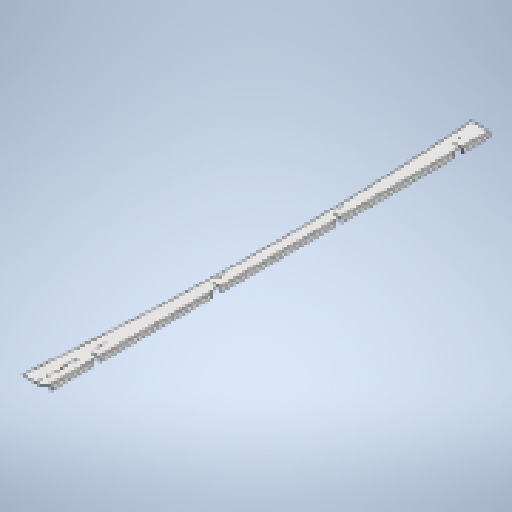
# Autodesk Inventor part: MSC 052 rib board_CPY
Saved by Autodesk Inventor 2025 (Build 290162010, 162A)
## iProperties
Created: 2024-04-28
Part Number: MSC 052 rib board_CPY
Material: Stainless Steel
Document SubType Name: Sheet Metal
Designer: admin
Stock Number: МОО 052 шпангоут борт
Density: 8 g/cm^3
Flat Pattern Width: 111.5 cm
Flat Pattern Length: 9.15826 cm
Flat Pattern Area: 1021.15 cm^2
Sheet Metal Rule: AISI304 2mm Die16
Sheet Metal Width: 1115,000 mm
Sheet Metal Length: 91,583 mm
Sheet Metal Area: 102114,551 mm^2
Appearance: Default
Author: admin
Стрингер_3: 67,524 mm
Стрингер_4: 48,201 mm
Стрингер_5: 51,522 mm
Стрингер_6: 77,509 mm
Autodesk Inventor part; units mm, degrees
note: some values were not read from the file. Chosen so that the rebuilt part matches the saved one: relief shape of "Plate4".
ref_plane "YZ Plane" through (0, 0, 0) normal (1, 0, 0) x (0, 1, 0)
ref_plane "XZ Plane" through (0, 0, 0) normal (0, 1, 0) x (-1, 0, 0)
ref_plane "XY Plane" through (0, 0, 0) normal (0, 0, 1) x (1, 0, 0)
sketch "Sketch1" plane through (0, 0, 0) normal (0, 0, 1) x (1, 0, 0)
  arc A0 (750, -2100) -> (770.156, -238.4205) centre (-10250, -1050) ccw construction
  arc A1 (752.9864, -2100.2851) -> (771.2831, -213.263) centre (-10246.9891, -1050.0292) ccw
  line L0 (-750, -2700) -> (-750, 0) construction
  line L1 (-800, 50) -> (-800, -2750) construction
  line L2 (-850, -2800) -> (-850, 100) construction
  line L3 (850, 100) -> (850, -2800)
  line L4 (800, -2750) -> (800, 50) construction
  line L5 (750, 0) -> (750, -2700) construction
  line L6 (770.156, -238.4205) -> (767.1641, -238.6409) construction
  line L7 (768.2917, -213.4901) -> (771.2831, -213.263) construction
  arc A2 (747.4657, -5.0326) -> (744.8748, -2.3426) centre (744.4792, -5.3164) ccw construction
  arc A3 (747.4657, -5.0326) -> (747.0136, -0.2851) centre (-10252.9895, -1050.2527) ccw construction
  arc A4 (767.1641, -238.6409) -> (747.4657, -5.0326) centre (-10252.9895, -1050.2527) ccw construction
  line L8 (750, 0) -> (747.0136, -0.2851) construction
  arc A5 (750.4522, -4.7486) -> (750, 0) centre (-10250, -1050) ccw construction
  arc A6 (750.4522, -4.7486) -> (745.2706, 0.6314) centre (744.4791, -5.3162) ccw
  line L9 (-750, 0) -> (750, 0) construction
  line L10 (-850, 100) -> (850, 100) construction
  line L11 (800, 50) -> (-800, 50) construction
  arc A7 (770.156, -238.4205) -> (750.4522, -4.7486) centre (-10250, -1050) ccw
  line L12 (750, -2700) -> (-750, -2700) construction
  line L13 (750, -2100) -> (752.9864, -2100.2851) construction
  line L14 (-800, -2750) -> (800, -2750)
  line L15 (850, -2800) -> (-850, -2800) construction
  arc A8 (110, -2700) -> (114.1118, -2698.3696) centre (110, -2694) ccw construction
  line L16 (0, -2697) -> (110, -2697) construction
  line L17 (0, -2700) -> (0, -2697) construction
  arc A9 (750, 0) -> (745.2706, 0.6314) centre (0, -5600) ccw construction
  line L18 (750, 0) -> (749.6018, -2.9735) construction
  arc A10 (750, -3.0268) -> (0, 47) centre (-0.2, -5603) ccw construction
  line L19 (0, 47) -> (0, 0) construction
  line L20 (0, 50) -> (0, 47) construction
  line L21 (0, 100) -> (0, 50)
  arc A11 (745.2706, 0.6314) -> (0, 50) centre (0, -5600) ccw construction
  line L22 (-750, -2100) -> (750, -2100) construction
  arc A12 (110, -2697) -> (112.0559, -2696.1848) centre (110, -2694) ccw construction
  line L23 (676.3163, -2173.4556) -> (674.2605, -2171.2708) construction
  line L24 (690.4112, -2151.9536) -> (692.4671, -2154.1384) construction
  line L25 (752.0559, -2102.1848) -> (676.3163, -2173.4556) construction
  line L26 (114.1118, -2698.3696) -> (750, -2100) construction
  arc A13 (752.0559, -2102.1848) -> (752.9864, -2100.2851) centre (749.9998, -2099.9999) ccw construction
  line L27 (750, -2100) -> (752.0559, -2102.1848) construction
  arc A14 (749.1768, -2100.7746) -> (750.1074, -2098.8746) centre (747.1209, -2098.5898) ccw construction
  line L28 (112.0559, -2696.1848) -> (690.4112, -2151.9536) construction
  line L29 (850, -258.4205) -> (774.6194, -258.4205)
  arc A15 (800, 50) -> (0, 100) centre (0, -6325) ccw construction
  arc A16 (824.6194, -258.4205) -> (800, 50) centre (-10711.2413, -1024.069) ccw construction
  line L30 (824.6194, -258.4205) -> (824.6194, 100) construction
  arc A17 (789.8132, -2131.1922) -> (824.6194, -258.4205) centre (-10201.1223, -990.2118) ccw construction
  line L31 (0, -2700) -> (0, -2750) construction
  line L32 (112.3791, -2700) -> (132.2053, -2750) construction
  line L33 (132.2053, -2750) -> (850, -2074.5565)
  arc A18 (770.0996, -238.4247) -> (766.3709, -188.564) centre (768.2917, -213.4901) ccw construction
  line L34 (850, -400) -> (783.8749, -400) construction
  line L35 (850, -900) -> (801.9923, -900) construction
  line L36 (850, -1400) -> (797.4674, -1400) construction
  line L37 (850, -1900) -> (770.2723, -1900) construction
  line L38 (350, 100) -> (350, 39.1489)
  line L39 (-1472.612, -150) -> (-973.4947, -150)
  line L40 (-1472.612, -700) -> (-973.4947, -700)
  line L41 (-1472.612, -1250) -> (-973.4947, -1250)
  line L42 (-1472.612, -1800) -> (-973.4947, -1800)
  line L43 (800, -2750) -> (850, -2750) construction
  line L44 (753.1643, -2098.4205) -> (850, -2098.4205)
  point P0 (824.6397, -2098.4205)
  dimension "d16" = 1500
  dimension "d17" = 2700
  dimension "d18" = 2100
  dimension "d19" = 6
  dimension "d20" = 3
  dimension "d21" = 3
  dimension "d22" = 6
  dimension "d23" = 3
  dimension "d24" = 239.271
  dimension "d25" = 50
  dimension "d26" = 50
  dimension "d27" = 3
  dimension "d28" = 110
  dimension "d29" = 25
  dimension "d30" = 104
  dimension "d31" = 25
  dimension "d32" = 20
  dimension "d33" = 50
  dimension "d57" = 500
  dimension "d58" = 500
  dimension "d59" = 500
  dimension "d60" = 500
  dimension "d61" = 500
  dimension "d83" = 250
  dimension "d86" = 550
  dimension "d91" = 274.5565
  dimension "d103" = 1.873
  dimension "d116" = 1840
  measures "d16" distance of L0.end L5.start
  measures "d17" distance of L5.start L5.end
  measures "d18" distance between parallel lines of L22 L9
  measures "d19" radius of A6
  measures "d20" radius of A2
  measures "d21" radius of A14
  measures "d22" radius of A8
  measures "d23" radius of A12
  measures "d24" distance of L6.start L5.start
  measures "d25" distance between parallel lines of L11 L10
  measures "d26" distance between parallel lines of L9 L11
  measures "d27" distance of L21.end L19.start
  measures "d28" distance from line of L17 A8.centre
  measures "d29" distance of L23.end L24.end
  measures "d30" distance of L27.start L23.end
  measures "d31" distance of L6.start L7.start
  measures "d32" vertical distance of L6.start L29.end
  measures "d33" distance of L30.start L29.end
  measures "d57" distance between parallel lines of L34 L10
  measures "d58" distance between parallel lines of L35 L34
  measures "d59" distance between parallel lines of L35 L36
  measures "d60" distance between parallel lines of L36 L37
  measures "d83" distance between parallel lines of L39 L10
  measures "d86" distance of L39.start L40.start
  measures "d91" distance from line of L33.end L42
  measures "d103" distance of L44.start L13.end
  measures "d116" distance between parallel lines of L44 L29
extrude "Plate3" add sketch "Sketch1" along normal blind 2 contours A1 L29 L3 L33 L44
sketch "Sketch3" plane through (848, -258.4205, 2) normal (1, 0, 0) x (0, 1, 0)
  line L0 (-1816.136, 0) -> (0, 0)
  line L1 (0, 0) -> (0, 20)
  line L2 (0, 20) -> (-1816.136, 20)
  line L3 (-1816.136, 20) -> (-1816.136, 0)
  constraints: 6 end point, 1 horizontal, 1 perpendicular, 1 vertical
edge flange "Flange2" height 20 angle 90 thickness 2 bend radius 2.75 thickness toward (1, 0, 0) relief tear relief width 2 relief depth 1 edges at (850, -1166.4885, 2) wall of the first edge with corners at (848, -2074.5565, 2) (848, -258.4205, 2) (848, -258.4205, -18) (848, -2074.5565, -18)
bend "Bend2"
corner "Corner2"
sketch "Sketch5" plane through (0, 0, 0) normal (0, 0, 1) x (1, 0, 0)
  line L0 (845.25, -2079.0263) -> (845.25, -258.4205) projected
  line L1 (774.6194, -258.4205) -> (845.25, -258.4205) projected
  arc A0 (753.1643, -2098.4205) -> (774.6194, -258.4205) centre (-10246.9891, -1050.0292) ccw projected
  line L2 (850, -258.4205) -> (850, -2074.5565) projected
  line L3 (850, -373.4205) -> (818, -373.4205)
  line L4 (850, -375.4205) -> (848, -375.4205) construction
  line L5 (848, -2074.5565) -> (848, -258.4205) projected
  line L6 (818, -373.4205) -> (818, -375.4205)
  line L7 (850, -873.4195) -> (801.5994, -873.4195) construction
  line L8 (850, -875.4195) -> (801.6312, -875.4195) construction
  line L9 (819, -873.4195) -> (819, -875.4195) construction
  line L10 (850, -1373.4195) -> (798.2777, -1373.4195) construction
  line L11 (850, -1375.4195) -> (798.2189, -1375.4195) construction
  line L12 (819, -1373.4195) -> (819, -1375.4195) construction
  line L13 (850, -1873.4195) -> (772.2907, -1873.4195) construction
  line L14 (850, -1875.4195) -> (772.1411, -1875.4195) construction
  line L15 (819, -1873.4195) -> (819, -1875.4195) construction
  line L16 (850, -904.4195) -> (845.25, -904.4195) construction
  line L17 (845.25, -1404.4195) -> (850, -1404.4195) construction
  line L18 (845.25, -1904.4195) -> (850, -1904.4195) construction
  line L19 (824.6397, -2098.4205) -> (753.1643, -2098.4205) projected
  line L20 (850, -373.4205) -> (850, -404.4205)
  line L21 (848, -373.4205) -> (848, -375.4205) construction
  line L22 (850, -404.4205) -> (848, -404.4205)
  line L23 (818, -373.4205) -> (782.2765, -373.4205) construction
  line L24 (818, -375.4205) -> (782.399, -375.4205) construction
  line L25 (848, -375.4205) -> (848, -404.4205)
  line L26 (848, -375.4205) -> (818, -375.4205)
  line L27 (848, -404.4205) -> (845.25, -404.4205)
  line L28 (845.25, -2079.0263) -> (824.6397, -2098.4205) projected
  point P0 (0, 0)
  point P1 (845.25, -380.4205)
  point P2 (848, -380.4205)
  point P3 (848, -1904.4195)
  point P4 (848, -1875.4195)
  point P5 (848, -1404.4195)
  point P6 (848, -1375.4195)
  point P7 (848, -904.4195)
  point P8 (848, -875.4195)
  point P9 (818, -374.4205)
  point P10 (848, -404.4205)
  point P11 (850, -410.4205)
  point P12 (848, -373.4205)
  point P13 (819, -874.4195)
  point P14 (819, -1374.4195)
  point P15 (819, -1874.4195)
  point P16 (848, -404.4205)
  point P17 (845.25, -375.4205)
  dimension "d69" = 1816.136
  dimension "d70" = 2
  dimension "d76" = 67.7235
  dimension "d80" = 48.4006
  dimension "d81" = 31
  dimension "d94" = 31
  dimension "d95" = 31
  dimension "d96" = 31
  dimension "d97" = 31
  dimension "d98" = 31
  dimension "d102" = 77.7093
  dimension "d104" = 51.7223
  dimension "d106" = 2
  dimension "d107" = 31
  dimension "d108" = 116
  dimension "d109" = 500
  dimension "d110" = 500
  dimension "d111" = 500
  dimension "d112" = 32
  constraints: 46 end point, 14 perpendicular, 13 point on line, 7 horizontal, 4 midpoint, 3 equal length, 3 parallel, 2 vertical, 22 other
  measures "d69" distance of point (850, -258.421) point (850, -2074.557)
  measures "d70" distance between parallel lines of L4 L3
  measures "d76" distance of L3.start L23.end
  measures "d80" distance of L7.start L7.end
  measures "d94" distance of L16.start L7.start
  measures "d95" distance of L12.start L10.start
  measures "d96" distance of L17.end L10.start
  measures "d97" distance of L15.start L13.start
  measures "d98" distance of L18.end L13.start
  measures "d102" distance of L13.start L13.end
  measures "d104" distance of L10.end L10.start
  measures "d106" distance of L22.end L20.end
  measures "d107" distance of L20.end L3.start
  measures "d108" vertical distance of point (850, -258.421) point (818, -374.421)
  measures "d109" distance of point (819, -874.42) point (818, -374.421)
  measures "d110" distance of point (819, -1374.42) point (819, -874.42)
  measures "d111" distance of point (819, -1874.42) point (819, -1374.42)
  measures "d112" distance of L3.end L3.start
extrude "Extrusion2" cut sketch "Sketch5" along normal through all both and the other way through all contours L0 L26 L5 L27 | L26 L6 L3 L0 | L0 L3 L5 L26 | L5 L3 L2 L22
chamfer "Chamfer2" distance 8 angle 45 1 edges at (845.25, -375.4205, 1)
pattern_linear "Rectangular Pattern3" count 4 spacing 500 along (0, -1, 0) of "Extrusion2", "Chamfer2"
sketch "Sketch6" plane through (0, 0, 0) normal (0, 0, -1) x (-1, 0, 0)
  line L0 (-803.1643, -2093.4205) -> (-815.1643, -2093.4205) construction
  line L1 (-815.1643, -2093.4205) -> (-815.1643, -1893.4205) construction
  line L2 (-815.1643, -1893.4205) -> (-803.1643, -1893.4205) construction
  line L3 (-803.1643, -1893.4205) -> (-803.1643, -2093.4205) construction
  line L4 (-753.1643, -2098.4205) -> (-824.6397, -2098.4205) projected
  line L5 (-803.1643, -1798.4205) -> (-803.1643, -1848.4205) construction
  line L6 (-803.1643, -1848.4205) -> (-815.1643, -1848.4205) construction
  line L7 (-815.1643, -1848.4205) -> (-815.1643, -1798.4205) construction
  line L8 (-815.1643, -1798.4205) -> (-803.1643, -1798.4205) construction
  line L9 (-845.25, -1873.4205) -> (-818, -1873.4205) projected
  line L10 (-803.1643, -1298.4205) -> (-803.1643, -1348.4205) construction
  line L11 (-803.1643, -1348.4205) -> (-815.1643, -1348.4205) construction
  line L12 (-815.1643, -1348.4205) -> (-815.1643, -1298.4205) construction
  line L13 (-815.1643, -1298.4205) -> (-803.1643, -1298.4205) construction
  line L14 (-803.1643, -798.4205) -> (-803.1643, -848.4205) construction
  line L15 (-803.1643, -848.4205) -> (-815.1643, -848.4205) construction
  line L16 (-815.1643, -848.4205) -> (-815.1643, -798.4205) construction
  line L17 (-815.1643, -798.4205) -> (-803.1643, -798.4205) construction
  line L18 (-803.1643, -298.4205) -> (-803.1643, -348.4205) construction
  line L19 (-803.1643, -348.4205) -> (-815.1643, -348.4205) construction
  line L20 (-815.1643, -348.4205) -> (-815.1643, -298.4205) construction
  line L21 (-815.1643, -298.4205) -> (-803.1643, -298.4205) construction
  line L22 (-845.25, -1373.4205) -> (-818, -1373.4205) projected
  line L23 (-845.25, -873.4205) -> (-818, -873.4205) projected
  line L24 (-845.25, -373.4205) -> (-818, -373.4205) projected
  point P0 (0, 0)
  dimension "d120" = 200
  dimension "d121" = 12
  dimension "d123" = 5
  dimension "d124" = 50
  dimension "d125" = 12
  dimension "d126" = 50
  dimension "d127" = 25
  dimension "d128" = 50
  dimension "d129" = 12
  dimension "d130" = 50
  dimension "d131" = 12
  dimension "d132" = 50
  dimension "d133" = 12
  dimension "d134" = 50
  dimension "d135" = 25
  dimension "d136" = 25
  dimension "d137" = 25
  dimension "d138" = 50
  dimension "d139" = 50
  dimension "d140" = 50
  constraints: 10 other
  measures "d120" distance of L0.end L1.end
  measures "d121" distance of L1.end L2.end
  measures "d123" distance between parallel lines of L4 L0
  measures "d124" horizontal distance of L4.start L0.start
  measures "d125" distance of L7.end L5.start
  measures "d126" distance of L6.end L7.end
  measures "d127" distance between parallel lines of L9 L6
  measures "d128" horizontal distance of L4.start L5.end
  measures "d129" distance of L13.start L13.end
  measures "d130" distance of L11.end L13.start
  measures "d131" distance of L17.start L17.end
  measures "d132" distance of L15.end L17.start
  measures "d133" distance of L21.start L21.end
  measures "d134" distance of L19.end L21.start
  measures "d135" distance between parallel lines of L22 L11
  measures "d136" distance between parallel lines of L23 L15
  measures "d137" distance between parallel lines of L24 L19
  measures "d138" horizontal distance of L4.start L10.end
  measures "d139" horizontal distance of L4.start L14.end
  measures "d140" horizontal distance of L4.start L18.end
mark "Mark1"
sketch "Sketch7" plane through (0, 0, 0) normal (0, 0, 1) x (1, 0, 0)
  line L0 (837.25, -1875.4205) -> (845.25, -1883.4205) construction
  line L1 (837.25, -1875.4205) -> (818, -1875.4205) construction
  line L2 (818, -1875.4205) -> (818, -1873.4205) construction
  line L3 (818, -1873.4205) -> (845.25, -1873.4205) construction
  line L4 (845.25, -1873.4205) -> (845.25, -1404.4205) construction
  line L5 (845.25, -1404.4205) -> (845.25, -1383.4205) construction
  line L6 (837.25, -1375.4205) -> (845.25, -1383.4205) construction
  line L7 (837.25, -1375.4205) -> (818, -1375.4205) construction
  line L8 (818, -1375.4205) -> (818, -1373.4205) construction
  line L9 (818, -1373.4205) -> (845.25, -1373.4205) construction
  line L10 (845.25, -1373.4205) -> (845.25, -904.4205) construction
  line L11 (845.25, -904.4205) -> (845.25, -883.4205) construction
  line L12 (837.25, -875.4205) -> (845.25, -883.4205) construction
  line L13 (837.25, -875.4205) -> (818, -875.4205) construction
  line L14 (818, -875.4205) -> (818, -873.4205) construction
  line L15 (818, -873.4205) -> (845.25, -873.4205) construction
  line L16 (845.25, -873.4205) -> (845.25, -404.4205) construction
  line L17 (845.25, -404.4205) -> (845.25, -383.4205) projected
  line L18 (837.25, -375.4205) -> (845.25, -383.4205) projected
  line L19 (837.25, -375.4205) -> (818, -375.4205) projected
  line L20 (818, -375.4205) -> (818, -373.4205) projected
  line L21 (818, -373.4205) -> (845.25, -373.4205) projected
  line L22 (845.25, -373.4205) -> (845.25, -258.4205) projected
  line L23 (774.6194, -258.4205) -> (845.25, -258.4205) projected
  arc A0 (753.1643, -2098.4205) -> (774.6194, -258.4205) centre (-10246.9891, -1050.0292) ccw construction
  line L24 (824.6397, -2098.4205) -> (753.1643, -2098.4205) construction
  line L25 (845.25, -2079.0263) -> (824.6397, -2098.4205) construction
  line L26 (845.25, -2079.0263) -> (845.25, -1904.4205) construction
  line L27 (845.25, -1904.4205) -> (845.25, -1883.4205) construction
  line L28 (716.6808, -2129.5736) -> (990.5996, -2129.5736)
  line L29 (990.5996, -2129.5736) -> (990.5996, -1373.4205)
  line L30 (990.5996, -1373.4205) -> (716.6808, -1373.4205)
  line L31 (716.6808, -1373.4205) -> (716.6808, -2129.5736)
  point P0 (0, 0)
  constraints: 8 end point, 2 parallel, 1 collinear, 1 horizontal, 1 perpendicular
extrude "Extrusion3" cut sketch "Sketch7" along normal through all both and the other way through all
equation "\"d16\" = d34"
equation "\"d17\" = d35"
equation "\"d18\" = d36"
equation "\"d19\" = d37"
equation "\"d20\" = d38"
equation "\"d21\" = d39"
equation "\"d22\" = d39 + d43"
equation "\"d23\" = d39"
equation "\"d24\" = d40"
equation "\"d27\" = d39"
equation "\"d28\" = 0.5 * d44"
equation "\"d29\" = d41"
equation "\"d30\" = d42"
equation "\"d31\" = d41"
equation "\"d33\" = d25"
equation "\"Стрингер_3\" = 67.5235"
equation "\"d37\" = d39 + d43"
equation "\"d38\" = d39"
equation "\"d43\" = d39"
equation "\"Стрингер_4\" = 48.20059"
equation "\"Стрингер_5\" = 51.52235"
equation "\"Стрингер_6\" = 77.5093"
equation "\"d34\" = 1500"
equation "\"d35\" = 2700"
equation "\"d36\" = 2100"
equation "\"d39\" = 3"
equation "\"d40\" = 239.271"
equation "\"d44\" = 220"
equation "\"d41\" = 25"
equation "\"d42\" = 104"
body "Solid2"
